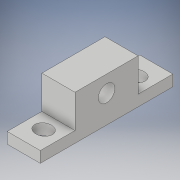
# Autodesk Inventor part: SuperiorBancada
Saved by Autodesk Inventor 2019 (Build 230136000, 136)
## iProperties
Created: 2019-07-02
Part Number: SuperiorBancada
Material: Generic
Document SubType Name: Modeling
Designer: Oscar Rojas
Density: 1 g/cm^3
Appearance: Default
Mass: 9.25971 g
Surface Area: 40.8039 cm^2
Volume: 9.25971 cm^3
Author: Oscar Rojas
Autodesk Inventor part; units mm, degrees
ref_plane "YZ Plane" through (0, 0, 0) normal (1, 0, 0) x (0, 1, 0)
ref_plane "XZ Plane" through (0, 0, 0) normal (0, 1, 0) x (-1, 0, 0)
ref_plane "XY Plane" through (0, 0, 0) normal (0, 0, 1) x (1, 0, 0)
sketch "Sketch1" plane through (0, 0, 0) normal (0, 1, 0) x (-1, 0, 0)
  line L0 (0, 0) -> (-20, 0)
  line L1 (-20, 0) -> (-20, -60)
  line L2 (-20, -60) -> (0, -60)
  line L3 (0, -60) -> (0, 0)
  line L4 (0, -60) -> (-15, -60)
  line L5 (0, -60) -> (15, -60) construction
  line L6 (-15, -60) -> (-15, 0)
  dimension "d0" = 20
  dimension "d1" = 60
  dimension "d14" = 15
  dimension "d15" = 180
  constraints: 14 end point, 2 collinear, 2 horizontal, 2 parallel, 2 perpendicular, 1 point on line
  measures "d0" distance of L2.end L1.end
  measures "d1" distance of L1.end L0.end
  measures "d14" distance of L2.end L4.end
  measures "d15" angle of L4 L5
extrude "Extrusion1" add sketch "Sketch1" along normal blind 5
sketch "Sketch2" plane through (0, 5, 0) normal (0, 1, 0) x (1, 0, 0)
  line L0 (10, 0) -> (19, 0) construction
  line L1 (0, 0) -> (20, 0) projected
  line L2 (0, 0) -> (15, 0) construction
  line L3 (7.5, 0) -> (16.5, 0) construction
  line L4 (0, 60) -> (0, 0) construction
  line L5 (7.5, 9) -> (0, 9) construction
  circle A0 centre (7.5, 51) radius 0.425 construction
  line L6 (7.5, 51) -> (1.0192, 51) construction
  line L7 (7.5, 51) -> (7.5, 47.5) construction
  line L8 (7.5, 51) -> (11.5, 51) construction
  ellipse E0 centre (7.5, 51) end of major axis (11.5, 51) minor radius 3.5
  line L9 (20, 0) -> (20, 60) construction
  line L10 (20, 30) -> (0, 30) construction
  ellipse E1 centre (7.5, 9) end of major axis (11.5, 9) minor radius 3.5
  dimension "d30" = 0.85
  dimension "d32" = 3.5
  dimension "d33" = 4
  constraints: 16 end point, 6 horizontal, 2 midpoint, 1 centre point, 1 coincident, 1 perpendicular, 1 point on line, 1 symmetric about line, 1 vertical, 6 other
  measures "d30" diameter of A0
  measures "d32" distance of L6.start L7.end
  measures "d33" distance of L6.start L8.end
sketch "Sketch3" plane through (0, 5, 0) normal (0, 1, 0) x (1, 0, 0)
  line L0 (0, 60) -> (0, 0) projected
  line L1 (20, 0) -> (20, 60) projected
  line L2 (0, 15.7197) -> (20, 15.7197)
  line L3 (20, 15.7197) -> (20, 44.2851)
  line L4 (20, 44.2851) -> (0, 44.2851)
  line L5 (0, 44.2851) -> (0, 15.7197)
  constraints: 8 end point, 2 parallel, 2 point on line, 1 horizontal, 1 perpendicular
extrude "Extrusion3" add sketch "Sketch3" along normal blind 15
sketch "Sketch4" plane through (20, 0, 0) normal (1, 0, 0) x (0, 0, -1)
  line L0 (15.7197, 5) -> (15.7197, 20) projected
  line L1 (44.2851, 5) -> (60, 5) projected
  circle A0 centre (30.0024, 12.5) radius 3.75
  point P0 (0, 0)
  dimension "d11" = 7.5
  constraints: 1 centre point
  measures "d11" diameter of A0
extrude "Extrusion4" cut sketch "Sketch4" against normal blind 65.5
extrude "Extrusion5" add sketch "Sketch1" along normal blind 5 contours L3 L2 L6 L0
extrude "Extrusion6" cut sketch "Sketch1" along normal blind 22.5 contours L6 L2 L1 L0
extrude "Extrusion9" cut sketch "Sketch2" against normal blind 10
body "Solid1"
